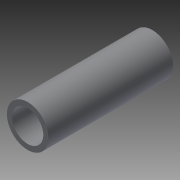
# Autodesk Inventor part: 52008.43
Saved by Autodesk Inventor 2014 SP2 (Build 180246200, 246)
## iProperties
Created: 2018-12-09
Part Number: 52008.43
Material: Generic
Catalog Web Link: www.cadenas.de
Description: SP-Spanner
Vendor: COLSONGROUP
Document SubType Name: Modeling
Designer: psadmin
Manufacturer: COLSONGROUP
Mass: 2.11155 g
Surface Area: 27.7106 cm^2
Volume: 2.11155 cm^3
Density: 1 g/cm^3
Appearance: PSOLRGB-175-175-175
Category: PARTsolutions
Company: COLSONGROUP
Title: 52008.43
Author: Cadenas PARTsolutions
Comments: Spanner
PSOL_IDENT_0: {$CADENAS_DATA\23d-libs\colsongroup\colson\wheels\accessories\colson_spanner.prj},153 {VTYP=3D},{NB=
PSOL_IDENT_1: 52008.43},{LINA=52008.43},{NN=SP},{DATE=25.04.2017 08:54:01},{GEOMDATE=15.12.2016 11:52:30},{VERSION=
PSOL_IDENT_2: },{LINEID=140},{WBVAR=},{WBNUMERIC=}  {NB=52008.43},{LINA=52008.43},{KT=DUMMY},{PN=52008.43},{ID=0.3
PSOL_IDENT_3: 75},{OD=0.5000},{L=1.5000},{OD2=0.659},{L2=0.41},{DD=1.5},{T=0.185}
NN: SP
NT: Spanner
NB: 52008.43
NBSYN: $PN.
LINA: 52008.43
PN: 52008.43
ID: 0.375
OD: 0.5
L: 1.5
SUPPLIER: COLSONGROUP
ARTICLENO: 52008.43
BOMINFO: 52008.43
CREATOR: CADENAS GmbH
Autodesk Inventor part; units mm, degrees
sketch "Sketch_1" plane through (0, 0, 0) normal (1, 0, 0) x (0, 1, 0)
  line L0 (0, -19.05) -> (0, 19.05)
  line L1 (4.7625, 19.05) -> (4.7625, -19.05)
  line L2 (4.7625, -19.05) -> (6.35, -19.05)
  line L3 (6.35, -19.05) -> (6.35, 19.05)
  line L4 (6.35, 19.05) -> (4.7625, 19.05)
  constraints: 10 end point
revolve "Revolution1" add sketch "Sketch_1" angle 360 about axis through (0, 0, -19.05) along (0, 0, -1)
ref_plane "spanner_XY" through (0, 0, 0) normal (0, 0, 1) x (1, 0, 0)
ref_plane "spanner_YZ" through (0, 0, 0) normal (1, 0, 0) x (0, 1, 0)
ref_plane "spanner_ZX" through (0, 0, 0) normal (0, 1, 0) x (0, 0, 1)
body "Solid1"
